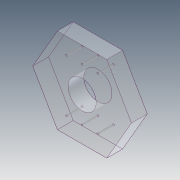
# Autodesk Inventor part: JF-AT-TM0009
Saved by Autodesk Inventor 2015 SP1 (Build 190203100, 203)
## iProperties
Created: 2010-04-06
Part Number: JF-AT-TM0009
Document SubType Name: Modeling
Designer: Osborne J.
Density: 0.66 g/cm^3
Material: Acrylic, Clear
Mass: 260.484 g
Surface Area: 459.54 cm^2
Volume: 394.672 cm^3
Description: 16 inch ball treadmill frame base v2
Appearance: Polycarbonate (Clear)
Revision Number: 0
Autodesk Inventor part; units mm, degrees
ref_plane "YZ Plane" through (0, 0, 0) normal (1, 0, 0) x (0, 1, 0)
ref_plane "XZ Plane" through (0, 0, 0) normal (0, 1, 0) x (-1, 0, 0)
ref_plane "XY Plane" through (0, 0, 0) normal (0, 0, 1) x (1, 0, 0)
sketch "Sketch1" plane through (0, 0, 0) normal (0, 0, 1) x (1, 0, 0)
  line L0 (44.45, -76.9897) -> (-44.45, -76.9897)
  line L1 (-44.45, -76.9897) -> (-88.9, 0)
  line L2 (-88.9, 0) -> (-44.45, 76.9897)
  line L3 (-44.45, 76.9897) -> (44.45, 76.9897)
  line L4 (44.45, 76.9897) -> (88.9, 0)
  line L5 (88.9, 0) -> (44.45, -76.9897)
  circle A0 centre (0, 0) radius 25.4
  line L6 (0, 107.7855) -> (0, -107.7855) projected
  line L7 (-124.46, 0) -> (124.46, 0) projected
  point P0 (0, 0)
  point P1 (0, 0)
  dimension "d1" = 88.9
  dimension "d4" = 50.8
  dimension "d7" = 88.9
  dimension "d8" = 88.9
  dimension "d9" = 88.9
  dimension "d10" = 120
  dimension "d11" = 120
  dimension "d12" = 120
  dimension "d13" = 120
  dimension "d14" = 120
  dimension "d15" = 44.45
  constraints: 12 end point, 1 centre point, 1 coincident, 1 symmetric about line, 14 other
  measures "d1" distance of L0.end L1.end
  measures "d4" diameter of A0
  measures "d7" distance of L2.end L3.end
  measures "d8" distance of L1.end L2.end
  measures "d9" distance of L3.end L4.end
  measures "d10" angle of L3 L2
  measures "d11" angle of L5 L4
  measures "d12" angle of L4 L3
  measures "d13" angle of L2 L1
  measures "d14" angle of L0 L1
  measures "d15" distance from line of L2.end L6
extrude "Extrusion1" add sketch "Sketch1" along normal blind 28.448
sketch "Sketch2" plane through (0, 0, 0) normal (0, 0, -1) x (-1, 0, 0)
  line L0 (-44.45, -76.9897) -> (44.45, -76.9897) projected
  line L1 (44.45, -76.9897) -> (88.9, 0) projected
  line L2 (88.9, 0) -> (44.45, 76.9897) projected
  line L3 (44.45, 76.9897) -> (-44.45, 76.9897) projected
  line L4 (-44.45, 76.9897) -> (-88.9, 0) projected
  line L5 (-88.9, 0) -> (-44.45, -76.9897) projected
  circle A0 centre (0, 0) radius 25.4 projected
  point P0 (0, 0)
  point P1 (0, 0)
  constraints: 1 coincident
extrude "Extrusion2" cut sketch "Sketch1" along normal blind 44.45 contours L6 L7 A0 | A0 L7 L6 | L7 L6 A0 | A0 L6 L7
sketch "Sketch3" plane through (0, 0, 28.448) normal (0, 0, 1) x (1, 0, 0)
  line L0 (0, 107.7855) -> (0, -107.7855) projected
  line L1 (-124.46, 0) -> (124.46, 0) projected
  line L2 (28.194, 47.244) -> (28.194, -47.244) construction
  line L3 (28.194, -47.244) -> (-28.194, -47.244) construction
  line L4 (-28.194, -47.244) -> (-28.194, 47.244) construction
  line L5 (-28.194, 47.244) -> (28.194, 47.244) construction
  line L6 (28.194, 47.244) -> (-28.194, -47.244) construction
  line L7 (28.194, -47.244) -> (-28.194, 47.244) construction
  point P0 (0, 0)
  point P1 (0, 47.244)
  point P2 (0, -47.244)
  dimension "d16" = 56.388
  dimension "d17" = 94.488
  dimension "d18" = 0
  constraints: 12 end point, 4 coincident, 4 midpoint, 2 parallel, 1 perpendicular
  measures "d16" distance of L2.end L3.end
  measures "d17" distance of L2.start L2.end
  measures "d18" angle of L0 L4
hole "Hole1" at (-28.194, 47.244, 28.448) at (28.194, 47.244, 28.448) at (28.194, -47.244, 28.448) at (-28.194, -47.244, 28.448) at (0, 47.244, 28.448) at (0, -47.244, 28.448) direction (0, 0, -1) diameter 3.302 end through all thread size "8-32 UNC" class "2B" standard "ANSI Unified Screw Threads"
body "Solid1"
